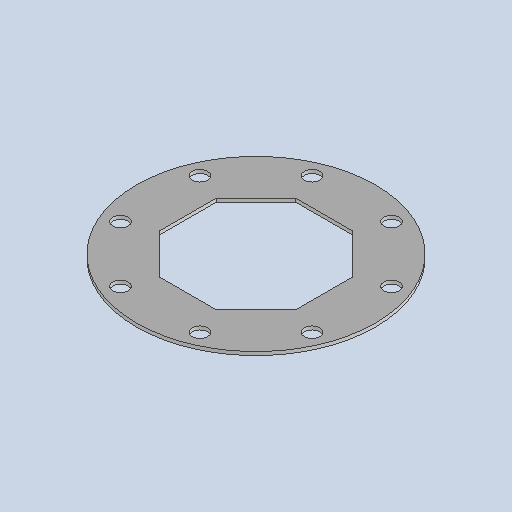
# Autodesk Inventor part: NDV-1103 Center flange 01
Saved by Autodesk Inventor 2026.2 (Build 302298000, 298)
## iProperties
Created: 2025-06-24
Part Number: NDV-1103 Center flange 01
Material: Stainless Steel
Document SubType Name: Sheet Metal
Designer: admin
Mass: 1869.22 g
Surface Area: 1641.67 cm^2
Volume: 233.653 cm^3
Density: 8 g/cm^3
Flat Pattern Width: 34 cm
Flat Pattern Length: 34 cm
Flat Pattern Area: 1156 cm^2
Sheet Metal Rule: Default
Sheet Metal Width: 340,000 mm
Sheet Metal Length: 340,000 mm
Sheet Metal Area: 115600,000 mm^2
Appearance: Default
Stock Number: Фланец центра нижний
Author: user
Autodesk Inventor part; units mm, degrees
ref_plane "YZ Plane" through (0, 0, 0) normal (1, 0, 0) x (0, 1, 0)
ref_plane "XZ Plane" through (0, 0, 0) normal (0, 1, 0) x (-1, 0, 0)
ref_plane "XY Plane" through (0, 0, 0) normal (0, 0, 1) x (1, 0, 0)
sketch "Sketch1" plane through (0, 0, 0) normal (0, 0, 1) x (1, 0, 0)
  circle A0 centre (0, 0) radius 170
  circle A1 centre (-56.4458, 136.2722) radius 11
  circle A2 centre (0, 0) radius 147.5 construction
  circle A3 centre (-136.2722, 56.4458) radius 11
  circle A4 centre (-136.2722, -56.4458) radius 11
  circle A5 centre (-56.4458, -136.2722) radius 11
  line L0 (40.1787, -97) -> (-40.1787, -97)
  line L1 (-40.1787, -97) -> (-97, -40.1787)
  line L2 (-97, -40.1787) -> (-97, 40.1787)
  line L3 (-97, 40.1787) -> (-40.1787, 97)
  line L4 (-40.1787, 97) -> (40.1787, 97)
  line L5 (40.1787, 97) -> (97, 40.1787)
  line L6 (97, 40.1787) -> (97, -40.1787)
  line L7 (97, -40.1787) -> (40.1787, -97)
  line L8 (0, 0) -> (-40.6608, 98.1639) construction
  circle A6 centre (56.4458, -136.2722) radius 11
  circle A7 centre (136.2722, -56.4458) radius 11
  circle A8 centre (136.2722, 56.4458) radius 11
  circle A9 centre (56.4458, 136.2722) radius 11
  dimension "d171" = 295
  dimension "d157" = 340
  dimension "d170" = 22
  dimension "d174" = 360
  dimension "d176" = 194
  dimension "d178" = 67.5
  measures "d157" diameter of A0
  measures "d170" diameter of A1
  measures "d176" distance between parallel lines of L4 L0
  measures "d178" angle of L8 L4
extrude "Plate5" add sketch "Sketch1" along normal blind 5
derived "NDV-0010 Parameters 01.ipt"
body "Solid3"
